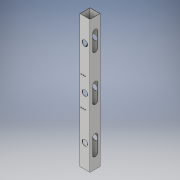
# Autodesk Inventor part: 2x2x26
Saved by Autodesk Inventor 2018 (Build 220112000, 112)
## iProperties
Created: 2018-01-17
Part Number: 2x2x26
Material: Generic
Document SubType Name: Modeling
Designer: S-2512711
Density: 1 g/cm^3
Appearance: Default
Author: S-2512711
Autodesk Inventor part; units mm, degrees
ref_plane "YZ Plane" through (0, 0, 0) normal (1, 0, 0) x (0, 1, 0)
ref_plane "XZ Plane" through (0, 0, 0) normal (0, 1, 0) x (-1, 0, 0)
ref_plane "XY Plane" through (0, 0, 0) normal (0, 0, 1) x (1, 0, 0)
sketch "Sketch1" plane through (0, 0, 0) normal (0, 1, 0) x (-1, 0, 0)
  line L0 (0, 0) -> (50.8, 0)
  line L1 (50.8, 0) -> (50.8, -50.8)
  line L2 (50.8, -50.8) -> (0, -50.8)
  line L3 (0, -50.8) -> (0, 0)
  line L4 (49.2125, -1.5875) -> (1.5875, -1.5875)
  line L5 (1.5875, -1.5875) -> (1.5875, -49.2125)
  line L6 (1.5875, -49.2125) -> (49.2125, -49.2125)
  line L7 (49.2125, -49.2125) -> (49.2125, -1.5875)
  dimension "d0" = 50.8
  dimension "d1" = 50.8
  dimension "d2" = 1.5875
  dimension "d3" = 1.5875
  dimension "d4" = 1.5875
  dimension "d5" = 1.5875
  constraints: 16 end point, 4 parallel, 2 horizontal, 2 perpendicular
  measures "d0" distance of L1.end L2.end
  measures "d1" distance of L0.end L1.end
  measures "d2" distance between parallel lines of L1 L7
  measures "d3" distance between parallel lines of L3 L5
  measures "d4" distance between parallel lines of L2 L6
  measures "d5" distance between parallel lines of L0 L4
extrude "Extrusion1" add sketch "Sketch1" along normal blind 660.4
sketch "Sketch2" plane through (-50.8, 0, 0) normal (0, 0, 1) x (1, 0, 0)
  line L0 (1.5875, 0) -> (49.2125, 0) projected
  line L1 (25.4, 0) -> (25.4, 660.4)
  line L2 (49.2125, 660.4) -> (1.5875, 660.4) projected
  line L3 (25.4, 0) -> (25.4, 104.775)
  line L4 (25.4, 660.4) -> (25.4, 555.625)
  circle A0 centre (25.4, 330.2) radius 14.2875
  line L5 (25.4, 330.2) -> (25.4, 115.2)
  line L6 (25.4, 330.2) -> (25.4, 545.2)
  circle A1 centre (25.4, 115.2) radius 14.2875
  circle A2 centre (25.4, 545.2) radius 14.2875
  point P0 (50.8, 0)
  dimension "d8" = 104.775
  dimension "d9" = 104.775
  dimension "d47" = 215
  dimension "d48" = 215
  constraints: 10 end point, 4 point on line, 3 centre point, 3 midpoint, 2 coincident
  measures "d8" distance of L1.start L3.end
  measures "d9" distance of L1.end L4.end
  measures "d47" distance of L5.start L5.end
  measures "d48" distance of L5.start L6.end
extrude "Extrusion2" cut sketch "Sketch2" against normal blind 530.225
sketch "Sketch3" plane through (-50.8, 0, 0) normal (0, 0, 1) x (1, 0, 0)
  circle A0 centre (25.4, 330.2) radius 14.2875 projected
  circle A1 centre (16.4338, 257.9624) radius 2.54
  line L0 (16.4338, 257.9624) -> (6.9088, 257.9624)
  line L1 (16.4338, 257.9624) -> (25.9588, 257.9624)
  circle A2 centre (6.9088, 257.9624) radius 2.54
  circle A3 centre (25.9588, 257.9624) radius 2.54
  circle A4 centre (16.4338, 402.4376) radius 2.54
  circle A5 centre (6.9088, 402.4376) radius 2.54
  circle A6 centre (25.9588, 402.4376) radius 2.54
  line L2 (50.8, 0) -> (50.8, 660.4) projected
  line L3 (25.4, 330.2) -> (25.4, 344.4875)
  line L4 (16.4338, 399.8976) -> (16.4338, 402.4376)
  line L5 (25.4, 330.2) -> (25.4, 315.9125)
  line L6 (16.4338, 260.5024) -> (16.4338, 257.9624)
  dimension "d15" = 5.08
  dimension "d16" = 9.525
  dimension "d17" = 9.525
  dimension "d49" = 24.8412
  dimension "d50" = 9.525
  dimension "d51" = 9.525
  dimension "d52" = 72.2376
  dimension "d53" = 24.8412
  dimension "d54" = 72.2376
  constraints: 12 end point, 4 centre point, 4 coincident, 4 vertical, 2 horizontal, 2 point on circle, 2 vertical alignment, 4 other
  measures "d16" distance of L0.start L0.end
  measures "d17" distance of L0.start L1.end
  measures "d49" distance from line of L2 A6.centre
  measures "d50" distance of L4.end A6.centre
  measures "d51" distance of L4.end A5.centre
  measures "d52" vertical distance of A6.centre L3.start
  measures "d53" distance from line of L2 L1.end
  measures "d54" vertical distance of L3.start L1.end
extrude "Extrusion3" cut sketch "Sketch3" against normal blind 101.6 contours L1 L6 A1 | A1 L0 L1 | L6 L0 A1 | A2 | A3 | A4 | A5 | A6
sketch "Sketch4" plane through (0, 0, 0) normal (1, 0, 0) x (0, 0, -1)
  circle A0 centre (25.4, 593.725) radius 12.7
  circle A1 centre (25.4, 517.525) radius 12.7
  line L0 (0, 660.4) -> (50.8, 660.4) projected
  line L1 (50.8, 0) -> (50.8, 660.4) projected
  line L2 (12.7, 593.725) -> (12.7, 517.525)
  line L3 (38.1, 517.525) -> (38.1, 593.725)
  point P0 (0, 0)
  dimension "d20" = 25.4
  dimension "d21" = 25.4
  dimension "d22" = 66.675
  dimension "d25" = 25.4
  dimension "d27" = 25.4
  dimension "d28" = 76.2
  constraints: 4 end point, 4 point on circle, 2 centre point, 2 tangent, 1 parallel, 1 vertical
  measures "d20" diameter of A0
  measures "d21" diameter of A1
  measures "d22" distance from line of A0.centre L0
  measures "d25" distance from line of L1 A0.centre
  measures "d27" distance from line of L1 A1.centre
  measures "d28" distance of A1.centre A0.centre
extrude "Extrusion4" cut sketch "Sketch4" against normal blind 127
sketch "Sketch5" plane through (0, 0, 0) normal (1, 0, 0) x (0, 0, -1)
  circle A0 centre (25.4, 66.675) radius 12.7
  circle A1 centre (25.4, 142.875) radius 12.7
  line L0 (50.8, 0) -> (0, 0) projected
  line L1 (0, 0) -> (0, 660.4) projected
  line L2 (50.8, 0) -> (50.8, 660.4) projected
  line L3 (12.7, 142.875) -> (12.7, 66.675)
  line L4 (38.1, 142.875) -> (38.1, 66.675)
  dimension "d31" = 25.4
  dimension "d32" = 25.4
  dimension "d33" = 66.675
  dimension "d34" = 25.4
  dimension "d35" = 25.4
  dimension "d36" = 76.2
  constraints: 4 end point, 4 point on circle, 2 centre point, 1 parallel, 1 tangent, 1 vertical
  measures "d31" diameter of A0
  measures "d32" diameter of A1
  measures "d33" distance from line of A0.centre L0
  measures "d34" distance from line of L1 A0.centre
  measures "d35" distance from line of L2 A1.centre
  measures "d36" distance of A0.centre A1.centre
extrude "Extrusion5" cut sketch "Sketch5" against normal blind 127
sketch "Sketch6" plane through (0, 0, 0) normal (1, 0, 0) x (0, 0, -1)
  circle A0 centre (25.4, 292.1) radius 12.7
  circle A1 centre (25.4, 368.3) radius 12.7
  line L0 (50.8, 0) -> (50.8, 660.4) projected
  line L1 (0, 0) -> (0, 660.4) projected
  line L2 (50.8, 0) -> (0, 0) projected
  line L3 (12.7, 368.3) -> (12.7, 292.1)
  line L4 (38.1, 368.3) -> (38.1, 292.1)
  dimension "d39" = 25.4
  dimension "d40" = 25.4
  dimension "d41" = 25.4
  dimension "d42" = 25.4
  dimension "d43" = 292.1
  dimension "d44" = 76.2
  constraints: 4 end point, 4 point on circle, 2 centre point, 2 tangent, 1 parallel, 1 vertical
  measures "d39" diameter of A0
  measures "d40" diameter of A1
  measures "d41" distance from line of L0 A1.centre
  measures "d42" distance from line of L1 A0.centre
  measures "d43" distance from line of L2 A0.centre
  measures "d44" distance of A0.centre A1.centre
extrude "Extrusion6" cut sketch "Sketch6" against normal blind 127
body "Solid1"
